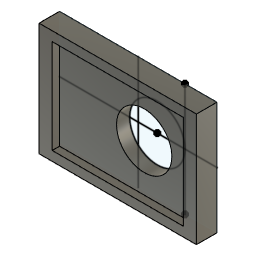
case (Autodesk Fusion 360 design; units mm, degrees)
Autodesk Fusion 360 part; units mm, degrees
box "BoxPrimitive1" add length 150 width 64 height 46 placed x (0, 1, 0) y (-1, 0, 0) z (0, 0, 1) at (4, 0, 0) makes body 1
sketch "Sketch3" plane through (0, 150, 0) normal (0, 1, 0) x (-1, 0, 0)
  line L0 (-4, 46) -> (-4, 0)
  line L1 (-4, 0) -> (60, 0)
  line L2 (60, 0) -> (60, 46)
  line L3 (60, 46) -> (-4, 46)
  line L4 (28, 46) -> (28, 0)
  line L5 (-4, 23) -> (60, 23)
  circle A0 centre (28, 23) radius 12.5
  dimension "d6" = 25
  constraint midpoint L3 L4.start
  constraint midpoint L1 L4.end
  constraint midpoint L0 L5.start
  constraint midpoint L2 L5.end
  constraint midpoint L5 A0.centre
  measures "d6" diameter of A0
copy_body "CopyPasteBodies1" bodies 1 makes body 2
scale "Scale1" factors (1.2, 1.1, 1.2) about (-60, 150, 46) bodies 2
sketch "Sketch6" plane through (0, 150, 0) normal (0, 1, 0) x (-1, 0, 0)
  line L0 (-16.8, 46) -> (-16.8, -9.2)
  line L1 (-16.8, -9.2) -> (60, -9.2)
  line L2 (60, -9.2) -> (60, 46)
  line L3 (60, 46) -> (-16.8, 46)
  line L4 (-16.8, 46) -> (60, -9.2)
  line L5 (60, 46) -> (-16.8, -9.2)
  point P0 (21.6, 18.4)
  constraint coincident L0.start L3.end
  constraint coincident L1.end L2.start
  constraint coincident L2.end L3.start
  constraint coincident L0.end L1.start
  constraint midpoint L5 P0
move_body "Move1" bodies 2 to x (1, 0, 0) y (0, 1, 0) z (0, 0, 1) at (-6.4, 0, 4.6)
move_body "Move2" bodies 2 to x (1, 0, 0) y (0, 1, 0) z (0, 0, 1) at (0, 6.4, 0)
extrude "Extrude1" add 1 faces at (-17.3333, 0, 15.3333) along direction (0, -1, 0) blind 25 on bodies 1 bodies 1
combine "Combine1" operation cut target body 2 tool bodies 1
sketch "Sketch7" plane through (0, 156.4, 0) normal (0, 1, 0) x (-1, 0, 0)
  line L0 (-10.4, 50.6) -> (-10.4, -4.6)
  line L1 (-10.4, -4.6) -> (66.4, -4.6)
  line L2 (66.4, -4.6) -> (66.4, 50.6)
  line L3 (66.4, 50.6) -> (-10.4, 50.6)
  line L4 (28, 50.6) -> (28, -4.6)
  line L5 (-10.4, 23) -> (66.4, 23)
  line L6 (5.2, 50.6) -> (5.2, -4.6)
  circle A0 centre (18.7, 23) radius 13.5
  dimension "d15" = 15.6
  dimension "d16" = 27
  constraint midpoint L3 L4.start
  constraint midpoint L1 L4.end
  constraint midpoint L0 L5.start
  constraint midpoint L2 L5.end
  constraint coincident L3 L6.start
  constraint coincident L1 L6.end
  constraint perpendicular L1 L6
  constraint tangent L6 A0
  constraint coincident L5 A0.centre
  measures "d15" distance of L0.start L6.start
  measures "d16" diameter of A0
extrude "Extrude3" cut sketch "Sketch7" against normal blind 10 contours L4 L5 A0 | L4 L5 A0 | L4 L5 A0 | L4 L5 A0 bodies 2
ref_plane "WorkPlane1" through (2.6, 146.4, 36.8) normal (0, 1, 0) x (-1, 0, 0)
split "Split1" by plane through (2.6, 146.4, 36.8) normal (0, 1, 0) bodies 2 makes body 3 at (-55, 156.4, 23)
hidden bodies 2
equation "d15 = 9.2 mm + 6.4 mm"
